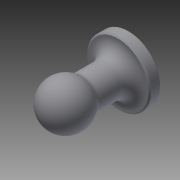
# Autodesk Inventor part: vertebro_front
Saved by Autodesk Inventor 2015 (Build 190159000, 159)
## iProperties
Created: 2014-11-07
Part Number: vertebro_front
Material: Generic
Document SubType Name: Modeling
Designer: Ryan
Density: 1 g/cm^3
Appearance: Default
Author: Ryan
Autodesk Inventor part; units mm, degrees
ref_plane "YZ Plane" through (0, 0, 0) normal (1, 0, 0) x (0, 1, 0)
ref_plane "XZ Plane" through (0, 0, 0) normal (0, 1, 0) x (-1, 0, 0)
ref_plane "XY Plane" through (0, 0, 0) normal (0, 0, 1) x (1, 0, 0)
sketch "Sketch1" plane through (0, 0, 0) normal (1, 0, 0) x (0, 1, 0)
  arc A0 (6.2933, 18.7067) -> (0, 33.9) centre (0, 25) ccw
  line L0 (0, 0) -> (12.5, 0)
  line L1 (12.5, 0) -> (12.5, 4.5)
  line L2 (12.5, 4.5) -> (6.2933, 4.5)
  line L3 (6.2933, 4.5) -> (6.2933, 18.7067)
  line L4 (0, 0) -> (0, 33.9)
  line L5 (0, 25) -> (6.2933, 18.7067) construction
  dimension "d0" = 17.8
  dimension "d1" = 12.5
  dimension "d2" = 25
  dimension "d3" = 4.5
  dimension "d5" = 45
  constraints: 12 end point, 3 perpendicular, 2 point on circle, 1 centre point, 1 horizontal, 1 parallel, 1 vertical alignment
  measures "d0" diameter of A0
  measures "d1" distance between parallel lines of L4 L1
  measures "d2" distance from line of L5.start L0
  measures "d3" distance between parallel lines of L0 L2
  measures "d5" angle of L4 L5
revolve "Revolution1" add sketch "Sketch1" angle 360 about axis through (0, 0, 0) along (0, 0, 1)
fillet "Fillet1" radius 5 1 edges at (0, -6.2933, 4.5)
fillet "Fillet2" radius 3 1 edges at (0, -6.2933, 18.7067)
chamfer "Chamfer1" distance 0.5 angle 45 1 edges at (0, -12.5, 0)
chamfer "Chamfer2" distance 0.5 angle 45 1 edges at (0, -12.5, 4.5)
hole "Hole1" at (0, 0, 0) direction (0, 0, 1) diameter 3 depth 10 tip angle 118
sketch "Sketch2" plane through (0, 0, 0) normal (0, 0, -1) x (-1, 0, 0)
  line L0 (0, 0) -> (-2.8865, 0)
  line L1 (0, 0) -> (0, -4.5)
  line L2 (-3.5, -4.5) -> (3.5, -4.5)
  line L3 (3.5, -4.5) -> (3.5, -6.5)
  line L4 (3.5, -6.5) -> (-3.5, -6.5)
  line L5 (-3.5, -6.5) -> (-3.5, -4.5)
  line L6 (-3.5, 4.5) -> (-3.5, 6.5)
  line L7 (-3.5, 6.5) -> (3.5, 6.5)
  line L8 (3.5, 6.5) -> (3.5, 4.5)
  line L9 (3.5, 4.5) -> (-3.5, 4.5)
  dimension "d23" = 4.5
  dimension "d24" = 2
  dimension "d25" = 7
  constraints: 20 end point, 6 perpendicular, 2 horizontal, 2 vertical, 1 midpoint, 1 symmetric about line, 4 other
  measures "d23" distance of L0.start L1.end
  measures "d24" distance of L2.end L3.end
  measures "d25" distance of L3.end L4.end
extrude "Extrusion1" add sketch "Sketch2" along normal blind 3
body "Solid1"
